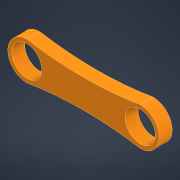
# Autodesk Inventor part: 04_Ramię-1
Saved by Autodesk Inventor 2022 (Build 260153000, 153)
## iProperties
Created: 2022-05-07
Part Number: 04_Ramię-1
Material: Generic
Document SubType Name: Modeling
Designer: pzach
Density: 1 g/cm^3
Appearance: Orange
Author: pzach
Autodesk Inventor part; units mm, degrees
ref_plane "YZ Plane" through (0, 0, 0) normal (1, 0, 0) x (0, 1, 0)
ref_plane "XZ Plane" through (0, 0, 0) normal (0, 1, 0) x (-1, 0, 0)
ref_plane "XY Plane" through (0, 0, 0) normal (0, 0, 1) x (1, 0, 0)
sketch "Sketch1" plane through (0, 0, 0) normal (0, 0, 1) x (1, 0, 0)
  arc A0 (155.0242, 475.3604) -> (155.0242, -475.3604) centre (0, 0) ccw
  arc A1 (2844.9758, -475.3604) -> (2844.9758, 475.3604) centre (3000, 0) ccw
  arc A2 (0, 500) -> (3000, 500) centre (1500, 9437.5) ccw
  line L0 (0, 0) -> (3000, 0) construction
  arc A3 (3000, -500) -> (0, -500) centre (1500, -9437.5) ccw
  circle A4 centre (0, 0) radius 400
  circle A5 centre (3000, 0) radius 400
  point P0 (0, -500)
  point P1 (3000, -500)
  dimension "d0" = 1000
  dimension "d1" = 1000
  dimension "d2" = 3000
  dimension "d4" = 9062.5
  dimension "d5" = 9437.5
  dimension "d6" = 500
  dimension "d7" = 800
  dimension "d8" = 800
  constraints: 14 point on circle, 6 centre point, 3 coincident, 3 symmetric about line, 2 end point, 1 horizontal, 1 horizontal alignment, 1 other
  measures "d0" diameter of A0
  measures "d1" diameter of A1
  measures "d2" distance of L0.start L0.end
  measures "d4" radius of A2
  measures "d5" distance from line of L0 A2.centre
  measures "d6" distance from line of A2.end L0
  measures "d7" diameter of A4
  measures "d8" diameter of A5
extrude "Extrusion1" add sketch "Sketch1" along normal mid plane 344.901 contours A2 A1 A3 A0
body "Solid1"
